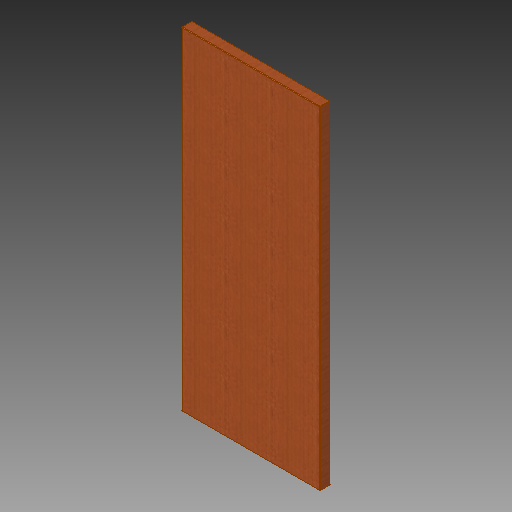
# Autodesk Inventor part: 2125_Wood Bench Top_V1
Saved by Autodesk Inventor 2020 (Build 240168000, 168)
## iProperties
Created: 2019-10-13
Part Number: 2125_Wood Bench Top_V1
Material: Oak, Red
Document SubType Name: Modeling
Designer: RFLab
Density: 0.673 g/cm^3
Appearance: Cherry - Natural Low Gloss
Mass: 53584.7 g
Surface Area: 30695.7 cm^2
Volume: 79620.7 cm^3
Author: RFLab
Autodesk Inventor part; units mm, degrees
ref_plane "YZ Plane" through (0, 0, 0) normal (1, 0, 0) x (0, 1, 0)
ref_plane "XZ Plane" through (0, 0, 0) normal (0, 1, 0) x (-1, 0, 0)
ref_plane "XY Plane" through (0, 0, 0) normal (0, 0, 1) x (1, 0, 0)
sketch "Sketch1" plane through (0, 0, 0) normal (0, 0, 1) x (1, 0, 0)
  line L0 (-381, -914.4) -> (381, -914.4)
  line L1 (381, -914.4) -> (381, 914.4)
  line L2 (381, 914.4) -> (-381, 914.4)
  line L3 (-381, 914.4) -> (-381, -914.4)
  line L4 (-381, -914.4) -> (381, 914.4) construction
  line L5 (381, -914.4) -> (-381, 914.4) construction
  point P0 (0, 0)
  dimension "d0" = 762
  dimension "d1" = 1828.8
  constraints: 12 end point, 2 midpoint, 2 parallel, 1 horizontal, 1 perpendicular
  measures "d0" distance of L2.end L1.end
  measures "d1" distance of L1.end L0.end
extrude "Extrusion1" add sketch "Sketch1" along normal mid plane 57.15
fillet "Fillet1" radius 3 12 edges at (0, -914.4, 28.575) (381, -914.4, 0) (381, 0, 28.575) (381, 914.4, 0) (0, 914.4, 28.575) (-381, 914.4, 0) (-381, 0, 28.575) (-381, -914.4, 0) (381, 0, -28.575) (0, 914.4, -28.575) (-381, 0, -28.575) (0, -914.4, -28.575)
body "Solid1"
